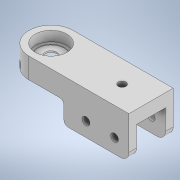
# Autodesk Inventor part: elbow joint 2
Saved by Autodesk Inventor 2022 (Build 260153000, 153)
## iProperties
Created: 2022-03-10
Part Number: elbow joint 2
Material: Genérico
Document SubType Name: Modeling
Designer: JK
Density: 1 g/cm^3
Appearance: Valor por defecto
Author: JK
Autodesk Inventor part; units mm, degrees
ref_plane "YZ Plane" through (0, 0, 0) normal (1, 0, 0) x (0, 1, 0)
ref_plane "XZ Plane" through (0, 0, 0) normal (0, 1, 0) x (-1, 0, 0)
ref_plane "XY Plane" through (0, 0, 0) normal (0, 0, 1) x (1, 0, 0)
sketch "Boceto1" plane through (0, 0, 0) normal (0, 1, 0) x (-1, 0, 0)
  circle A0 centre (0, 0) radius 12.625
  circle A1 centre (0, 0) radius 15.5
  dimension "d0" = 25.25
  dimension "d1" = 31
  constraints: 2 centre point, 2 coincident
  measures "d0" diameter of A0
  measures "d1" diameter of A1
extrude "Extrusión1" add sketch "Boceto1" along normal blind 6
sketch "Boceto2" plane through (0, 6, 0) normal (0, 1, 0) x (1, 0, 0)
  circle A0 centre (0, 0) radius 15.5 projected
  circle A1 centre (0, 0) radius 4.15
  dimension "d4" = 8.3
  constraints: 1 centre point, 1 coincident
  measures "d4" diameter of A1
extrude "Extrusión2" add sketch "Boceto2" along normal blind 1
sketch "Boceto3" plane through (0, 7, 0) normal (0, 1, 0) x (1, 0, 0)
  circle A0 centre (0, 0) radius 15.5 projected
  circle A1 centre (0, 0) radius 11.125
  dimension "d7" = 22.25
  constraints: 1 centre point, 1 coincident
  measures "d7" diameter of A1
extrude "Extrusión3" add sketch "Boceto3" along normal blind 7.5
sketch "Boceto4" plane through (0, 7, 0) normal (0, 1, 0) x (1, 0, 0)
  circle A0 centre (0, 0) radius 9.125
  circle A1 centre (0, 0) radius 11.125 projected
  dimension "d10" = 2
  constraints: 1 centre point, 1 coincident
  measures "d10" radial gap between concentric circles of A1 A0
extrude "Extrusión4" add sketch "Boceto4" along normal blind 0.5
sketch "Boceto5" plane through (0, 0, 0) normal (1, 0, 0) x (0, 1, 0)
  circle A0 centre (3, 0) radius 2.15
  line L0 (0, -15.5) -> (0, 15.5) projected
  point P0 (0, 0)
  dimension "d13" = 4.3
  dimension "d14" = 3
  constraints: 1 centre point
  measures "d13" diameter of A0
  measures "d14" distance from line of L0 A0.centre
extrude "Extrusión5" cut sketch "Boceto5" against normal through all
pattern_circular "Patrón circular1" count 3 over 102 about axis through (0, 6, 0) along (0, 1, 0) of "Extrusión5" both ways yes
sketch "Boceto6" plane through (0, 0, 0) normal (0, -1, 0) x (1, 0, 0)
  line L0 (-12.4406, 2.15) -> (-15.3502, 2.15) projected
  line L1 (-12.4406, -2.15) -> (-15.3502, -2.15) projected
  circle A0 centre (0, 0) radius 4.15 projected
  circle A1 centre (0, 0) radius 12.625 projected
  circle A2 centre (0, 0) radius 15.5 projected
  circle A3 centre (0, 0) radius 12.625 projected
extrude "Extrusión6" add sketch "Boceto6" against normal blind 7.5 contours A1 L1 A2 L0 picked at (-13.4651, 1.6733)
sketch "Boceto12" plane through (0, 14.5, 0) normal (0, 1, 0) x (1, 0, 0)
  line L0 (-70, 10) -> (70, 10)
  line L1 (70, 10) -> (70, -10)
  line L2 (70, -10) -> (-70, -10)
  line L3 (-70, -10) -> (-70, 10)
  circle A0 centre (0, 0) radius 4.15 projected
  line L4 (-70, 10) -> (70, -10) construction
  line L5 (70, 10) -> (-70, -10) construction
  line L6 (-70, 15.5) -> (70, 15.5)
  line L7 (70, 15.5) -> (70, -15.5)
  line L8 (70, -15.5) -> (-70, -15.5)
  line L9 (-70, -15.5) -> (-70, 15.5)
  line L10 (-70, 15.5) -> (70, -15.5) construction
  line L11 (70, 15.5) -> (-70, -15.5) construction
  circle A1 centre (0, 0) radius 15.5 projected
  circle A2 centre (0, 0) radius 17.5
  point P0 (11.8427, -10)
  point P1 (0, -15.5)
  point P2 (70, -10)
  point P3 (0, 15.5)
  point P4 (11.8427, 10)
  point P5 (70, 10)
  dimension "d39" = 140
  dimension "d40" = 20
  dimension "d43" = 35
  constraints: 24 end point, 4 midpoint, 4 parallel, 2 horizontal, 2 perpendicular, 1 centre point, 1 coincident, 1 collinear, 1 tangent
  measures "d39" distance of L1.end L2.end
  measures "d40" distance of L0.end L1.end
  measures "d43" diameter of A2
extrude "Extrusión11" add sketch "Boceto12" against normal up to surface (14.5 mm away) contours A1 L6 A2 L0 | L0 A2 L2 A1 | L6 L7 L0 A2 | L0 L1 L2 A2 | L2 A2 L8 A1 | A2 L2 L7 L8 picked at (11.2785, 11.4928) picked at (13.347, 8.995) picked at (11.2785, -11.4928)
sketch "Boceto13" plane through (0, 0, 0) normal (0, -1, 0) x (1, 0, 0)
  circle A0 centre (0, 0) radius 24.5
  circle A1 centre (0, 0) radius 12.625 projected
  arc A2 (0, 15.5) -> (0, -15.5) centre (0, 0) ccw projected
  line L0 (0, -15.5) -> (70, -15.5) projected
  line L1 (70, -15.5) -> (70, 15.5) projected
  line L2 (70, 15.5) -> (0, 15.5) projected
  line L3 (70, 15.5) -> (0, 15.5) projected
  line L4 (24.5, 15.5) -> (24.5, -15.5)
  line L5 (70, -15.5) -> (0, -15.5) projected
  dimension "d44" = 49
  constraints: 2 end point, 2 point on line, 1 centre point, 1 coincident, 1 perpendicular
  measures "d44" diameter of A0
extrude "Extrusión12" add sketch "Boceto13" along normal blind 15 contours L4 L2 L1 L0
sketch "Boceto14" plane through (0, -15, 0) normal (0, -1, 0) x (1, 0, 0)
  line L0 (110.5, -10.15) -> (29.5, -10.15)
  line L1 (29.5, -10.15) -> (29.5, 10.15)
  line L2 (29.5, 10.15) -> (110.5, 10.15)
  line L3 (110.5, 10.15) -> (110.5, -10.15)
  line L4 (70, 15.5) -> (70, -15.5) projected
  line L5 (110.5, -10.15) -> (29.5, 10.15) construction
  line L6 (29.5, -10.15) -> (110.5, 10.15) construction
  line L7 (24.5, 15.5) -> (24.5, -15.5) projected
  line L8 (70, 15.5) -> (24.5, 15.5) projected
  point P0 (0, 0)
  point P1 (70, 0)
  point P2 (70, -10.15)
  point P3 (70, 10.15)
  dimension "d47" = 5
  dimension "d49" = 20.3
  constraints: 12 end point, 3 midpoint, 2 parallel, 1 horizontal, 1 perpendicular
  measures "d47" distance between parallel lines of L1 L7
  measures "d49" distance of L2.end L0.start
extrude "Extrusión13" cut sketch "Boceto14" against normal through all contours L0 L1 L2 L4
sketch "Boceto15" plane through (29.5, -15, 10.15) normal (1, 0, 0) x (0, 0, -1)
  circle A0 centre (10.15, 10) radius 2.7
  line L0 (20.3, 0) -> (0, 0) projected
  point P0 (10.15, 15)
  dimension "d52" = 5.4
  dimension "d53" = 10
  constraints: 1 centre point
  measures "d52" diameter of A0
  measures "d53" distance from line of A0.centre L0
extrude "Extrusión14" cut sketch "Boceto15" against normal blind 12
sketch "Boceto16" plane through (24.5, 0, -15.5) normal (-1, 0, 0) x (0, 0, 1)
  circle A0 centre (15.5, -5) radius 2.7 projected
  circle A1 centre (15.5, -5) radius 4.65
  point P0 (15.5, 0)
  dimension "d56" = 9.3
  constraints: 1 centre point, 1 coincident
  measures "d56" diameter of A1
extrude "Extrusión15" cut sketch "Boceto16" against normal blind 2 contours A0 | A1
fillet "Empalme4" radius 3 1 edges at (24.5, 0, 0)
sketch "Boceto18" plane through (70, -15, -15.5) normal (1, 0, 0) x (0, 0, -1)
  line L0 (0, 29.5) -> (-31, 29.5) projected
  line L1 (-25.65, 29.5) -> (-5.35, 29.5)
  line L2 (-5.35, 29.5) -> (-5.35, 20.3)
  line L3 (-5.35, 20.3) -> (-25.65, 20.3)
  line L4 (-25.65, 20.3) -> (-25.65, 29.5)
  line L5 (-5.35, 29.5) -> (-5.35, 0) projected
  line L6 (-5.35, 0) -> (-25.65, 0) projected
  line L7 (-25.65, 0) -> (-25.65, 29.5) projected
  point P0 (-15.5, 15)
  dimension "d60" = 20.3
  constraints: 8 end point, 2 collinear, 2 parallel, 1 horizontal, 1 perpendicular, 1 point on line
  measures "d60" distance between parallel lines of L3 L6
extrude "Extrusión16" add sketch "Boceto18" against normal up to surface (40.5 mm away) contours L2 L3 L4 L0
sketch "Boceto19" plane through (0, 14.5, 15.5) normal (0, 0, 1) x (1, 0, 0)
  circle A0 centre (40, -19.5) radius 2.7
  circle A1 centre (60, -19.5) radius 2.7
  line L0 (70, -29.5) -> (24.5, -29.5) projected
  line L1 (70, 0) -> (70, -29.5) projected
  point P0 (0, -14.5)
  dimension "d63" = 10
  dimension "d64" = 10
  dimension "d65" = 5.4
  dimension "d66" = 10
  dimension "d67" = 20
  constraints: 2 centre point, 1 equal radius
  measures "d63" distance from line of A0.centre L0
  measures "d64" distance from line of L0 A1.centre
  measures "d65" diameter of A0
  measures "d66" distance from line of L1 A1.centre
  measures "d67" distance of A1.centre A0.centre
extrude "Extrusión17" cut sketch "Boceto19" against normal through all
sketch "Boceto20" plane through (70, 5.3, -10.15) normal (0, -1, 0) x (1, 0, 0)
  circle A0 centre (-20.25, 10.15) radius 2.7
  point P0 (-70, 10.15)
  dimension "d70" = 5.4
  constraints: 1 centre point
  measures "d70" diameter of A0
extrude "Extrusión18" cut sketch "Boceto20" against normal through all
fillet "Empalme5" radius 6 2 edges at (70, -15, 12.825) (70, -15, -12.825)
fillet "Empalme6" radius 3 1 edges at (24.5, -15, 0)
sketch "Boceto7" plane through (0, 0, 0) normal (0, -1, 0) x (1, 0, 0)
  line L0 (50, 10.15) -> (-50, 10.15)
  line L1 (-50, 10.15) -> (-50, -10.15)
  line L2 (-50, -10.15) -> (50, -10.15)
  line L3 (50, -10.15) -> (50, 10.15)
  circle A0 centre (0, 0) radius 4.15 projected
  line L4 (50, 10.15) -> (-50, -10.15) construction
  line L5 (-50, 10.15) -> (50, -10.15) construction
  line L6 (-50, 15.5) -> (50, 15.5)
  line L7 (50, 15.5) -> (50, -15.5)
  line L8 (50, -15.5) -> (-50, -15.5)
  line L9 (-50, -15.5) -> (-50, 15.5)
  line L10 (-50, 15.5) -> (50, -15.5) construction
  line L11 (50, 15.5) -> (-50, -15.5) construction
  circle A1 centre (0, 0) radius 12.625 projected
  circle A2 centre (0, 0) radius 17.5 projected
  circle A3 centre (0, 0) radius 15.5 projected
  point P0 (14.2558, -10.15)
  point P1 (0, -17.5)
  point P2 (50, -10.15)
  point P3 (0, 17.5)
  point P4 (14.2558, 10.15)
  dimension "d22" = 20.3
  dimension "d23" = 50
  constraints: 24 end point, 4 midpoint, 4 parallel, 2 horizontal, 2 perpendicular, 1 collinear, 1 tangent
  measures "d22" distance between parallel lines of L2 L0
  measures "d23" distance from line of L3 point (0, 0)
sketch "Boceto8" plane through (0, 20, 0) normal (0, 1, 0) x (1, 0, 0)
  line L0 (0, -17.5) -> (50, -17.5) projected
  line L1 (17.5, -17.5) -> (17.5, 17.5)
  line L2 (50, 17.5) -> (0, 17.5) projected
  arc A0 (14.2558, -10.15) -> (14.2558, 10.15) centre (0, 0) ccw projected
  arc A1 (14.2558, -10.15) -> (14.2558, 10.15) centre (0, 0) ccw projected
  arc A2 (14.2558, 10.15) -> (0, 17.5) centre (0, 0) ccw projected
  arc A3 (0, 17.5) -> (0, -17.5) centre (0, 0) ccw projected
  arc A4 (0, -17.5) -> (14.2558, -10.15) centre (0, 0) ccw projected
  circle A5 centre (0, 0) radius 11.125 projected
  line L3 (50, 17.5) -> (0, 17.5) projected
  arc A6 (14.2558, 10.15) -> (0, 17.5) centre (0, 0) ccw projected
  line L4 (14.2558, 10.15) -> (50, 10.15) projected
  line L5 (50, 10.15) -> (50, 17.5) projected
  line L6 (50, -10.15) -> (14.2558, -10.15) projected
  arc A7 (0, -17.5) -> (14.2558, -10.15) centre (0, 0) ccw projected
  line L7 (0, -17.5) -> (50, -17.5) projected
  line L8 (50, -17.5) -> (50, -10.15) projected
  point P0 (17.5, -10.15)
  point P1 (17.5, 0)
  point P2 (17.5, 10.15)
  constraints: 2 end point, 2 point on line, 1 tangent, 1 vertical
sketch "Boceto9" plane through (0, 20, 0) normal (0, 1, 0) x (1, 0, 0)
  line L0 (0, 17.5) -> (50, 17.5) projected
  line L1 (50, -17.5) -> (0, -17.5) projected
  line L2 (0, 17.5) -> (0, -17.5)
  arc A0 (0, -17.5) -> (17.5, 0) centre (0, 0) ccw projected
  arc A1 (17.5, 0) -> (0, 17.5) centre (0, 0) ccw projected
  arc A2 (0, 17.5) -> (0, -17.5) centre (0, 0) ccw projected
  circle A3 centre (0, 0) radius 11.125 projected
  point P0 (0, 11.125)
  point P1 (0, -11.125)
  constraints: 2 end point, 1 vertical
sketch "Boceto11" plane through (0, 20, 0) normal (0, 1, 0) x (1, 0, 0)
  line L0 (50, -17.5) -> (0, -17.5) projected
  line L1 (16.2282, -17.5) -> (-27.539, -17.5)
  line L2 (-27.539, -17.5) -> (-27.539, 24.0171)
  line L3 (-27.539, 24.0171) -> (16.2282, 24.0171)
  line L4 (16.2282, 24.0171) -> (16.2282, -17.5)
  line L5 (17.5, -10.15) -> (17.5, 10.15) projected
  point P0 (0, 0)
  point P1 (0, -17.5)
  constraints: 8 end point, 2 parallel, 1 horizontal, 1 perpendicular, 1 point on line
